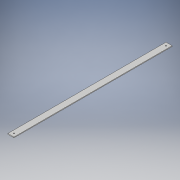
# Autodesk Inventor part: 1x1 24
Saved by Autodesk Inventor 2018 (Build 220112000, 112)
## iProperties
Created: 2018-06-29
Part Number: 1x1 24
Material: Generic
Document SubType Name: Modeling
Designer: s-2512711
Density: 1 g/cm^3
Appearance: Default
Author: s-2512711
Autodesk Inventor part; units mm, degrees
ref_plane "YZ Plane" through (0, 0, 0) normal (1, 0, 0) x (0, 1, 0)
ref_plane "XZ Plane" through (0, 0, 0) normal (0, 1, 0) x (-1, 0, 0)
ref_plane "XY Plane" through (0, 0, 0) normal (0, 0, 1) x (1, 0, 0)
sketch "Sketch1" plane through (0, 0, 0) normal (0, 0, 1) x (1, 0, 0)
  line L0 (0, 0) -> (25.4, 0)
  line L1 (25.4, 0) -> (25.4, 3.175)
  line L2 (25.4, 3.175) -> (0, 3.175)
  line L3 (0, 3.175) -> (0, 0)
  dimension "d23" = 25.4
  dimension "d24" = 3.175
  constraints: 8 end point, 2 parallel, 1 horizontal, 1 perpendicular
  measures "d23" distance of L2.end L1.end
  measures "d24" distance of L1.end L0.end
extrude "Extrusion1" add sketch "Sketch1" along normal blind 660.4
sketch "Sketch6" plane through (0, 3.175, 0) normal (0, 1, 0) x (1, 0, 0)
  line L0 (0, 0) -> (25.4, 0) projected
  line L1 (12.7, 0) -> (12.7, -12.7)
  line L2 (0, -660.4) -> (25.4, -660.4) projected
  line L3 (12.7, -660.4) -> (12.7, -647.7)
  circle A0 centre (12.7, -647.7) radius 2.5797
  circle A1 centre (12.7, -12.7) radius 2.5797
  dimension "d25" = 12.7
  dimension "d26" = 12.7
  dimension "d27" = 5.1594
  constraints: 4 end point, 2 centre point, 2 coincident, 2 midpoint, 2 vertical
  measures "d25" distance of L1.start L1.end
  measures "d26" distance of L3.start L3.end
  measures "d27" diameter of A0
extrude "Extrusion6" cut sketch "Sketch6" against normal blind 609.6
body "Solid1"
